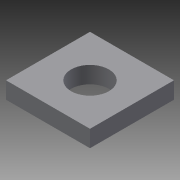
# Autodesk Inventor part: 1.25in Jig
Saved by Autodesk Inventor 2015 (Build 190159000, 159)
## iProperties
Created: 2015-02-14
Part Number: 1.25in Jig
Material: Generic
Document SubType Name: Modeling
Designer: robotics
Density: 1 g/cm^3
Appearance: Default
Author: robotics
Autodesk Inventor part; units mm, degrees
ref_plane "YZ Plane" through (0, 0, 0) normal (1, 0, 0) x (0, 1, 0)
ref_plane "XZ Plane" through (0, 0, 0) normal (0, 1, 0) x (-1, 0, 0)
ref_plane "XY Plane" through (0, 0, 0) normal (0, 0, 1) x (1, 0, 0)
sketch "Sketch1" plane through (0, 0, 0) normal (0, 1, 0) x (-1, 0, 0)
  circle A0 centre (0, 0) radius 28.5375
  line L0 (63.5, 63.5) -> (-63.5, 63.5)
  line L1 (-63.5, 63.5) -> (-63.5, -63.5)
  line L2 (-63.5, -63.5) -> (63.5, -63.5)
  line L3 (63.5, -63.5) -> (63.5, 63.5)
  dimension "d0" = 57.075
  dimension "d1" = 63.5
  dimension "d2" = 63.5
  dimension "d3" = 63.5
  dimension "d5" = 63.5
  constraints: 8 end point, 2 parallel, 1 centre point, 1 coincident, 1 horizontal, 1 perpendicular
  measures "d0" diameter of A0
  measures "d1" distance from line of L3 A0.centre
  measures "d2" distance from line of A0.centre L1
  measures "d3" distance from line of A0.centre L0
  measures "d5" distance from line of A0.centre L2
extrude "Extrusion1" add sketch "Sketch1" along normal blind 25.4
body "Solid1"
